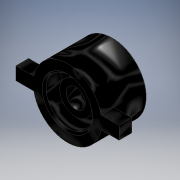
# Autodesk Inventor part: Button-SNES
Saved by Autodesk Inventor 2019 (Build 230136000, 136)
## iProperties
Created: 2018-06-05
Part Number: Button-SNES
Material: Plastique ABS
Document SubType Name: Modeling
Designer: dimercur
Density: 1.06 g/cm^3
Appearance: Noir
Author: dimercur
Autodesk Inventor part; units mm, degrees
ref_plane "YZ Plane" through (0, 0, 0) normal (1, 0, 0) x (0, 1, 0)
ref_plane "XZ Plane" through (0, 0, 0) normal (0, 1, 0) x (-1, 0, 0)
ref_plane "XY Plane" through (0, 0, 0) normal (0, 0, 1) x (1, 0, 0)
sketch "Esquisse1" plane through (0, 0, 0) normal (0, 1, 0) x (-1, 0, 0)
  circle A0 centre (0, 0) radius 5.3
  dimension "d0" = 10.6
  constraints: 1 centre point, 1 coincident
  measures "d0" diameter of A0
extrude "Extrusion1" add sketch "Esquisse1" along normal blind 7
shell "Coque2" thickness 1.7 removed faces 1 at (-1.6995, 0, -1.9343)
sketch "Esquisse6" plane through (0, 5.3, 0) normal (0, -1, 0) x (1, 0, 0)
  circle A0 centre (0, 0) radius 2.5
  circle A1 centre (0, 0) radius 1.5
  dimension "d20" = 5
  dimension "d21" = 3
  constraints: 2 centre point, 2 coincident
  measures "d20" diameter of A0
  measures "d21" diameter of A1
extrude "Extrusion4" add sketch "Esquisse6" along normal blind 4
sketch "Esquisse7" plane through (0, 0, 0) normal (0, -1, 0) x (1, 0, 0)
  line L0 (-8, 1) -> (-4.8, 1)
  line L1 (-4.8, 1) -> (-4.8, -1)
  line L2 (-4.8, -1) -> (-8, -1)
  line L3 (-8, -1) -> (-8, 1)
  line L4 (4.8, 1) -> (8, 1)
  line L5 (8, 1) -> (8, -1)
  line L6 (8, -1) -> (4.8, -1)
  line L7 (4.8, -1) -> (4.8, 1)
  point P0 (0, 0)
  dimension "d24" = 2
  dimension "d25" = 1
  dimension "d26" = 4.8
  dimension "d27" = 4.8
  dimension "d29" = 8
  dimension "d30" = 8
  constraints: 16 end point, 4 parallel, 2 horizontal, 2 perpendicular, 2 point on line
  measures "d24" distance of L2.end L0.start
  measures "d25" vertical distance of point (0, 0) L0.start
  measures "d26" distance from line of point (0, 0) L1
  measures "d27" distance from line of point (0, 0) L7
  measures "d29" distance from line of point (0, 0) L3
  measures "d30" distance from line of point (0, 0) L5
extrude "Extrusion5" add sketch "Esquisse7" against normal blind 2
fillet "Congé3" radius 0.1 1 edges at (5.3, 7, 0)
chamfer "Chanfrein1" distance 0.3 angle 45 1 edges at (3.6, 0, 0)
equation "\"d25\" = 0.5 * d24"
equation "\"d27\" = d26"
equation "\"d30\" = d29"
